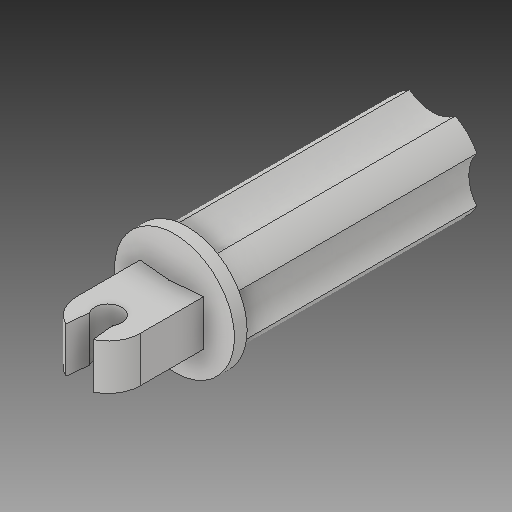
# Autodesk Inventor part: Top
Saved by Autodesk Inventor 2019 (Build 230136000, 136)
## iProperties
Created: 2019-03-03
Part Number: Top
Material: Generic
Document SubType Name: Modeling
Designer: alarr
Density: 1 g/cm^3
Appearance: Default
Author: alarr
Autodesk Inventor part; units mm, degrees
ref_plane "YZ Plane" through (0, 0, 0) normal (1, 0, 0) x (0, 1, 0)
ref_plane "XZ Plane" through (0, 0, 0) normal (0, 1, 0) x (-1, 0, 0)
ref_plane "XY Plane" through (0, 0, 0) normal (0, 0, 1) x (1, 0, 0)
sketch "Sketch1" plane through (0, 0, 0) normal (0, 0, 1) x (1, 0, 0)
  circle A0 centre (0, 0) radius 6.985
  dimension "d0" = 13.97
  constraints: 1 centre point, 1 coincident
  measures "d0" diameter of A0
extrude "Extrusion1" add sketch "Sketch1" against normal blind 34.29
sketch "Sketch2" plane through (0, 0, -34.29) normal (0, 0, -1) x (-1, 0, 0)
  circle A0 centre (0, 0) radius 1.7018
  dimension "d3" = 3.4036
  constraints: 1 centre point, 1 coincident
  measures "d3" diameter of A0
extrude "Extrusion2" cut sketch "Sketch2" against normal blind 36.322
sketch "Sketch3" plane through (0, 0, -34.29) normal (0, 0, -1) x (-1, 0, 0)
  circle A0 centre (0, 0) radius 6.985 projected
  arc A1 (-3.1957, 6.2111) -> (3.1957, 6.2111) centre (0, 10.16) ccw
  circle A2 centre (0, 0) radius 6.985 projected
  line L0 (0, 10.16) -> (0, 0) construction
  dimension "d6" = 10.16
  dimension "d7" = 5.08
  constraints: 4 point on circle, 2 end point, 1 centre point, 1 vertical
  measures "d6" distance of L0.start A0.centre
  measures "d7" radius of A1
extrude "Extrusion3" cut sketch "Sketch3" against normal through all contours A1 A0 picked at (-0.9288, 6.328)
pattern_circular "Circular Pattern1" count 4 over 360 about axis through (0, 0, -34.29) along (0, 0, 1) of "Extrusion3"
sketch "Sketch4" plane through (0, 0, 0) normal (0, 1, 0) x (-1, 0, 0)
  line L0 (0, 0) -> (8.382, 0)
  line L1 (8.382, 0) -> (8.382, 1.778)
  line L2 (8.382, 1.778) -> (0, 2.54)
  line L3 (0, 2.54) -> (0, 0)
  line L4 (-3.1957, 0) -> (3.1957, 0) projected
  line L5 (0, -41.656) -> (0, 9.906) projected
  dimension "d13" = 8.382
  dimension "d14" = 1.778
  dimension "d15" = 2.54
  constraints: 8 end point, 2 perpendicular, 1 horizontal
  measures "d13" distance between parallel lines of L3 L1
  measures "d14" distance of L0.end L1.end
  measures "d15" distance of L2.end L0.start
revolve "Revolution1" add sketch "Sketch4" angle 360 about axis through (0, 0, -10) along (0, 0, 1)
sketch "Sketch5" plane through (0, 0, 0) normal (0, 1, 0) x (-1, 0, 0)
  arc A0 (0, 6.5809) -> (4.445, 11.0259) centre (0, 11.0259) ccw construction
  line L0 (0, 2.54) -> (-8.382, 1.778) projected
  line L1 (0, 2.54) -> (8.382, 1.778) projected
  line L2 (0, 2.54) -> (0, 11.0259) construction
  line L3 (-4.445, 11.0259) -> (-4.445, 2.1359)
  line L4 (4.445, 11.0259) -> (4.445, 2.1359)
  arc A1 (-4.445, 11.0259) -> (0, 6.5809) centre (0, 11.0259) ccw construction
  arc A2 (4.445, 11.0259) -> (-4.445, 11.0259) centre (0, 11.0259) ccw
  point P0 (0, 0)
  dimension "d17" = 8.89
  dimension "d18" = 8.89
  constraints: 6 end point, 6 point on circle, 4 tangent, 3 centre point, 3 point on line, 3 vertical
  measures "d17" diameter of A0
  measures "d18" distance of L4.start L4.end
extrude "Extrusion4" add sketch "Sketch5" along normal mid plane 6.35
sketch "Sketch6" plane through (0, 3.175, 0) normal (0, 1, 0) x (1, 0, 0)
  arc A0 (-4.445, -11.0259) -> (4.445, -11.0259) centre (0, -11.0259) ccw projected
  arc A1 (1.5875, -12.0789) -> (-1.5875, -12.0789) centre (0, -11.0259) ccw
  line L0 (1.5875, -12.0789) -> (1.905, -15.042)
  line L1 (-1.5875, -12.0789) -> (-1.905, -15.042)
  arc A2 (-1.5875, -12.0789) -> (1.5875, -12.0789) centre (0, -11.0259) ccw construction
  line L2 (1.905, -15.042) -> (-1.905, -15.042) construction
  line L3 (1.5875, -12.0789) -> (-1.5875, -12.0789) construction
  point P0 (0, 0)
  dimension "d22" = 3.81
  dimension "d23" = 3.175
  dimension "d24" = 3.81
  constraints: 8 end point, 6 point on circle, 2 centre point, 2 horizontal, 1 coincident
  measures "d22" diameter of A1
  measures "d23" distance of L0.start L1.start
  measures "d24" distance of L0.end L1.end
extrude "Extrusion5" cut sketch "Sketch6" against normal through all
body "Solid1"
